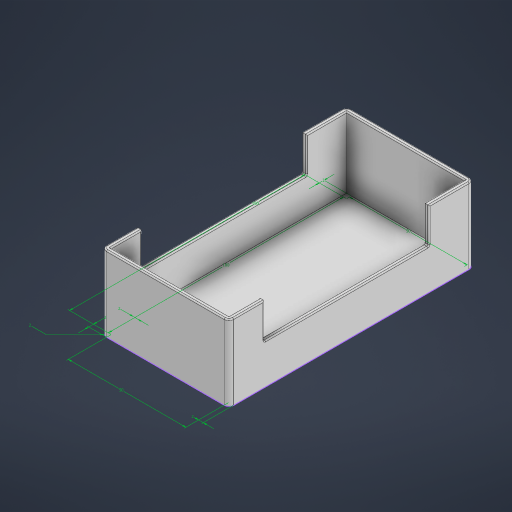
# Autodesk Inventor part: connection box
Saved by Autodesk Inventor 2024.2 (Build 282272000, 272)
## iProperties
Created: 2025-07-03
Part Number: connection box
Material: Generic
Document SubType Name: Modeling
Designer: Moe
Density: 1 g/cm^3
Appearance: Default
Author: Moe
Autodesk Inventor part; units mm, degrees
ref_plane "YZ Plane" through (0, 0, 0) normal (1, 0, 0) x (0, 1, 0)
ref_plane "XZ Plane" through (0, 0, 0) normal (0, 1, 0) x (-1, 0, 0)
ref_plane "XY Plane" through (0, 0, 0) normal (0, 0, 1) x (1, 0, 0)
sketch "Sketch1" plane through (0, 0, 0) normal (0, 1, 0) x (-1, 0, 0)
  line L0 (50, 2) -> (0, 2)
  line L1 (-2, 0) -> (-2, -100)
  line L2 (0, -102) -> (50, -102)
  line L3 (52, -100) -> (52, 0)
  arc A0 (52, 0) -> (50, 2) centre (50, 0) ccw
  arc A1 (0, 2) -> (-2, 0) centre (0, 0) ccw
  arc A2 (-2, -100) -> (0, -102) centre (0, -100) ccw
  arc A3 (50, -102) -> (52, -100) centre (50, -100) ccw
  line L4 (50, 0) -> (0, 0)
  line L5 (0, 0) -> (0, -100)
  line L6 (0, -100) -> (50, -100)
  line L7 (50, -100) -> (50, 0)
  point P0 (0, 0)
  point P1 (50, -100)
  point P2 (50, 0)
  point P3 (0, -100)
  dimension "d0" = 50
  dimension "d1" = 100
  dimension "d7" = 2
  dimension "d8" = 100
  dimension "d9" = 2
  dimension "d10" = 2
  dimension "d11" = 2
  dimension "d12" = 2
  dimension "d13" = 50
  constraints: 16 end point, 8 point on circle, 8 tangent, 4 centre point, 4 parallel, 3 equal radius, 2 horizontal, 2 perpendicular
  measures "d0" distance of point (50, -100) point (0, -100)
  measures "d1" distance of point (50, 0) point (50, -100)
  measures "d7" radius of A0
  measures "d8" distance between parallel lines of L6 L4
  measures "d9" distance between parallel lines of L2 L6
  measures "d10" distance between parallel lines of L0 L4
  measures "d11" distance between parallel lines of L3 L7
  measures "d12" distance between parallel lines of L1 L5
  measures "d13" distance of L4.start L4.end
extrude "Extrusion1" add sketch "Sketch1" along normal blind 2 contours A0 L3 A3 L2 A2 L1 A1 L0 | L7 L6 L5 L4
extrude "Extrusion2" add sketch "Sketch1" along normal blind 32
sketch "Sketch2" plane through (0, 32, 0) normal (0, 1, 0) x (1, 0, 0)
  arc A0 (0, -2) -> (2, 0) centre (0, 0) ccw projected
  line L0 (2, 0) -> (2, 100) projected
  arc A1 (2, 100) -> (0, 102) centre (0, 100) ccw projected
  line L1 (0, 102) -> (-50, 102) projected
  arc A2 (-50, 102) -> (-52, 100) centre (-50, 100) ccw projected
  line L2 (-52, 100) -> (-52, 0) projected
  arc A3 (-52, 0) -> (-50, -2) centre (-50, 0) ccw projected
  line L3 (-50, -2) -> (0, -2) projected
  line L4 (-50, 0) -> (-50, 100) projected
  line L5 (-50, 100) -> (0, 100) projected
  line L6 (0, 100) -> (0, 0) projected
  line L7 (0, 0) -> (-50, 0) projected
  line L8 (-50, 0) -> (0, 0) projected
  line L9 (0, 0) -> (0, 100) projected
  line L10 (0, 100) -> (-50, 100) projected
  line L11 (-50, 100) -> (-50, 0) projected
  line L12 (-52, 100) -> (-52, 0) projected
  line L13 (-52, 13) -> (-50, 13)
  line L14 (-50, 13) -> (-50, 83)
  line L15 (-50, 83) -> (-52, 83)
  line L16 (-52, 83) -> (-52, 13)
  line L17 (0, 13) -> (2, 13)
  line L18 (2, 13) -> (2, 83)
  line L19 (2, 83) -> (0, 83)
  line L20 (0, 83) -> (0, 13)
  point P0 (0, 0)
  point P1 (-52, 48)
  point P2 (0, 83)
  dimension "d18" = 2
  dimension "d19" = 70
  dimension "d20" = 50
  constraints: 16 end point, 4 parallel, 3 point on line, 2 horizontal, 2 perpendicular, 1 midpoint
  measures "d18" distance of L15.end L14.end
  measures "d19" distance of L14.end L13.end
  measures "d20" distance from line of L3 point (-52, 48)
extrude "Extrusion3" cut sketch "Sketch2" against normal blind 15 contours L17 L6 L19 L0 | L2 L15 L4 L13
fillet "Fillet1" radius 0.5 32 edges at (-52, 17, -48) (-50, 17, -48) (0, 17, -48) (2, 17, -48) (2, 24.5, -83) (0, 24.5, -83) (1, 17, -83) (1, 17, -13) (0, 24.5, -13) (2, 24.5, -13) (-50, 24.5, -83) (-52, 24.5, -83) (-51, 17, -83) (-50, 24.5, -13) (-52, 24.5, -13) (-51, 17, -13) (-50, 32, -91.5) (-51.4142, 32, -101.4142) (-25, 32, -102) (1.4142, 32, -101.4142) (2, 32, -91.5) (-52, 32, -91.5) (-25, 32, -100) (0, 32, -91.5) (1.4142, 32, 1.4142) (-25, 32, 2) (-51.4142, 32, 1.4142) (-52, 32, -6.5) (2, 32, -6.5) (0, 32, -6.5) (-25, 32, 0) (-50, 32, -6.5)
body "Solid1"
